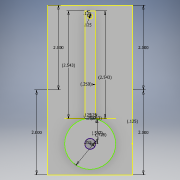
# Autodesk Inventor part: ClawLinkage
Saved by Autodesk Inventor 2017 (Build 210142000, 142)
## iProperties
Created: 2017-09-29
Part Number: ClawLinkage
Material: Generic
Document SubType Name: Modeling
Designer: User
Density: 1 g/cm^3
Appearance: Default
Author: User
Autodesk Inventor part; units mm, degrees
ref_plane "YZ Plane" through (0, 0, 0) normal (1, 0, 0) x (0, 1, 0)
ref_plane "XZ Plane" through (0, 0, 0) normal (0, 1, 0) x (-1, 0, 0)
sketch "Sketch1" plane through (0, 0, 0) normal (0, 0, 1) x (1, 0, 0)
  circle A0 centre (0, 0) radius 15.24
  constraints: 1 centre point
extrude "Extrusion1" add sketch "Sketch1" along normal blind 3.175
sketch "Sketch2" plane through (0, 0, 3.175) normal (0, 0, 1) x (1, 0, 0)
  circle A0 centre (0, 0) radius 15.24 projected
  line L0 (-15.24, 0) -> (-15.24, 3.175)
  line L1 (-15.24, 0) -> (-15.24, -3.175)
  dimension "d3" = 3.175
  dimension "d4" = 3.175
  constraints: 4 end point, 4 vertical, 1 horizontal alignment, 1 other
  measures "d3" distance of L0.start L0.end
  measures "d4" distance of L0.start L1.end
ref_plane "Work Plane1" through (-15.24, 0, 3.175) normal (1, 0, 0) x (0, 1, 0)
sketch "Sketch3" plane through (-15.24, 0, 3.175) normal (1, 0, 0) x (0, 1, 0)
  line L0 (15.24, 0) -> (-15.24, 0) projected
  line L1 (-15.24, -3.175) -> (15.24, -3.175) projected
  line L2 (0, -3.175) -> (3.175, -3.175)
  line L3 (3.175, -3.175) -> (3.175, 0)
  line L4 (3.175, 0) -> (-3.175, 0)
  line L5 (-3.175, 0) -> (-3.175, -3.175)
  line L6 (-3.175, -3.175) -> (3.175, -3.175)
  dimension "d6" = 6.35
  constraints: 10 end point, 3 perpendicular, 1 collinear, 1 point on line
  measures "d6" distance of L3.end L4.end
extrude "Extrusion2" add sketch "Sketch3" against normal blind 64.2493
sketch "Sketch4" plane through (-15.24, 0, 3.175) normal (1, 0, 0) x (0, 0, -1)
  line L0 (3.175, -3.175) -> (3.175, 0) projected
  line L1 (0, 3.175) -> (3.175, 3.175)
  line L2 (3.175, 3.175) -> (3.175, -3.175)
  line L3 (3.175, -3.175) -> (0, -3.175)
  line L4 (0, -3.175) -> (0, 3.175)
  constraints: 8 end point, 2 parallel, 1 horizontal, 1 perpendicular
extrude "Extrusion3" add sketch "Sketch4" along normal blind 12.7
sketch "Sketch6" plane through (0, 0, 0) normal (0, 0, -1) x (-1, 0, 0)
  circle A0 centre (0, 0) radius 3.2385
  dimension "d24" = 6.477
  constraints: 1 centre point, 1 coincident
  measures "d24" diameter of A0
hole "Hole1" at (0, 0, 0) direction (0, 0, -1) diameter 6.477 end through all
hole "Hole2" at (0, 0, 0) direction (0, 0, 1) diameter 6.477 depth 7.9375 tip angle 118
sketch "Sketch7" plane through (0, 0, 3.175) normal (0, 0, 1) x (1, 0, 0)
  line L0 (-79.4893, -3.175) -> (-79.4893, 3.175) projected
  line L1 (-79.4893, 0) -> (-76.3143, 0)
  circle A0 centre (-76.3143, 0) radius 1.5875
  point P0 (0, 0)
  dimension "d39" = 3.175
  dimension "d40" = 3.175
  constraints: 2 end point, 1 centre point, 1 coincident, 1 horizontal, 1 midpoint
  measures "d39" distance of L1.start L1.end
  measures "d40" diameter of A0
extrude "Extrusion6" cut sketch "Sketch7" against normal blind 25.4
sketch "Sketch8" plane through (0, 0, 3.175) normal (0, 0, 1) x (1, 0, 0)
  arc A0 (-14.9056, -3.175) -> (-14.9056, 3.175) centre (0, 0) ccw projected
  line L0 (-32.1247, -25.4) -> (18.6753, -25.4)
  line L1 (-32.1247, -25.4) -> (-82.9246, -25.4)
  line L2 (-32.1247, 25.4) -> (-82.9246, 25.4)
  line L3 (-32.1247, 25.4) -> (18.6753, 25.4)
  line L4 (18.6753, 25.4) -> (18.6753, -25.4)
  line L5 (-82.9246, 25.4) -> (-82.9246, -25.4)
  dimension "d45" = 50.8
  dimension "d46" = 50.8
  dimension "d47" = 50.8
  dimension "d48" = 50.8
  constraints: 12 end point, 3 horizontal
  measures "d45" distance of L0.start L0.end
  measures "d46" distance of L0.start L1.end
  measures "d47" distance of L2.start L2.end
  measures "d48" distance of L2.start L3.end
extrude "Extrusion7" add sketch "Sketch8" along normal blind 3.175
sketch "Sketch9" plane through (-79.4893, -3.175, 0) normal (0, -1, 0) x (1, 0, 0)
  line L0 (64.5837, 3.175) -> (64.5837, 0) projected
  line L1 (64.5837, 0) -> (64.5837, 3.175)
  point P0 (79.4893, 0)
  constraints: 2 end point, 1 collinear
sketch "Sketch10" plane through (-79.4893, 3.175, 0) normal (0, 1, 0) x (1, 0, 0)
  line L0 (64.5837, -3.175) -> (64.5837, 0) projected
  line L1 (64.5837, 0) -> (64.5837, -3.175)
  point P0 (79.4893, 0)
  constraints: 2 end point, 1 collinear
sketch "Sketch11" plane through (0, 0, 3.175) normal (0, 0, -1) x (-1, 0, 0)
  line L0 (14.9056, 3.175) -> (79.4893, 3.175) projected
  line L1 (79.4893, 3.175) -> (79.4893, -3.175) projected
  line L2 (14.9056, 3.175) -> (79.4893, 3.175)
  line L3 (79.4893, -3.175) -> (14.9056, -3.175) projected
  line L4 (14.9056, -3.175) -> (79.4893, -3.175)
  arc A0 (14.9056, 3.175) -> (14.9056, -3.175) centre (0, 0) ccw projected
  circle A1 centre (0, 0) radius 3.2385 projected
  line L5 (79.4893, -3.175) -> (14.9056, -3.175) projected
  dimension "d51" = 64.5837
  dimension "d52" = 64.5837
  dimension "d53" = 18.4785
  dimension "d54" = 6.35
  dimension "d55" = 14.9056
  constraints: 4 end point, 1 collinear, 1 perpendicular
  measures "d51" distance of L0.start L0.end
  measures "d52" distance of L1.end L3.end
  measures "d54" distance between parallel lines of L5 L0
  measures "d55" horizontal distance of L3.end A0.centre
sketch "Sketch12" plane through (-82.9246, -25.4, 3.175) normal (0, -1, 0) x (1, 0, 0)
  line L0 (0, 0) -> (101.6, 0) projected
  line L1 (68.019, -3.175) -> (98.1646, -3.175) projected
  point P0 (82.9246, -3.175)
  dimension "d56" = 3.175
  measures "d56" distance between parallel lines of L0 L1
sketch "Sketch13" plane through (0, 0, 3.175) normal (0, 0, -1) x (-1, 0, 0)
  point P0 (0, 0)
sketch "Sketch14" plane through (0, 0, 0) normal (0, 0, -1) x (-1, 0, 0)
  circle A0 centre (0, 0) radius 15.24 projected
  circle A1 centre (76.3143, 0) radius 1.5875 projected
  circle A2 centre (0, 0) radius 3.2385 projected
  line L0 (79.4893, -3.175) -> (14.9056, -3.175) projected
  line L1 (79.4893, 3.175) -> (79.4893, -3.175) projected
  line L2 (14.9056, 3.175) -> (79.4893, 3.175) projected
  arc A3 (14.9056, 3.175) -> (14.9056, -3.175) centre (0, 0) ccw projected
  line L3 (15.24, -15.24) -> (15.24, 15.24) projected
  line L4 (-18.6753, 25.4) -> (82.9246, 25.4) projected
  line L5 (-18.6753, -25.4) -> (-18.6753, 25.4) projected
  line L6 (82.9246, -25.4) -> (-18.6753, -25.4) projected
  line L7 (82.9246, 25.4) -> (82.9246, -25.4) projected
  line L8 (79.4893, 3.175) -> (14.9056, 3.175) projected
  line L9 (79.4893, -3.175) -> (79.4893, 3.175) projected
  line L10 (79.4893, -3.175) -> (14.9056, -3.175) projected
  arc A4 (14.9056, 3.175) -> (14.9056, -3.175) centre (0, 0) ccw projected
  line L11 (14.9056, -3.175) -> (14.9056, -3.5133)
  dimension "d57" = 0.3344
  constraints: 2 end point
  measures "d57" distance between parallel lines of L3 L11
body "Solid1"
